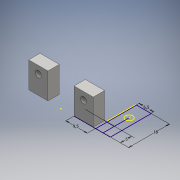
# Autodesk Inventor part: Part1
Saved by Autodesk Inventor 2016 (Build 200138000, 138)
## iProperties
Created: 2016-10-10
Part Number: Part1
Material: Generic
Document SubType Name: Modeling
Designer: yurra
Density: 1 g/cm^3
Appearance: Default
Author: yurra
Autodesk Inventor part; units mm, degrees
ref_plane "YZ Plane" through (0, 0, 0) normal (1, 0, 0) x (0, 1, 0)
ref_plane "XZ Plane" through (0, 0, 0) normal (0, 1, 0) x (-1, 0, 0)
sketch "Sketch1" plane through (0, 0, 0) normal (0, 1, 0) x (-1, 0, 0)
  line L0 (5.75, 3.75) -> (-5.75, 3.75)
  line L1 (-5.75, 3.75) -> (-5.75, -3.75)
  line L2 (-5.75, -3.75) -> (5.75, -3.75)
  line L3 (5.75, -3.75) -> (5.75, 3.75)
  line L4 (5.75, 3.75) -> (-5.75, -3.75) construction
  line L5 (-5.75, 3.75) -> (5.75, -3.75) construction
  line L6 (0, 0) -> (0, 3.75)
  circle A0 centre (10, 0.5) radius 1.25
  circle A1 centre (-10, 0.5) radius 1.25
  line L7 (8.328, 1.75) -> (12.3503, 1.75)
  line L8 (8.75, 3.0207) -> (8.75, -2.5964)
  line L9 (5.05, 3.25) -> (-5.05, 3.25)
  line L10 (-5.05, 3.25) -> (-5.05, -3.25)
  line L11 (-5.05, -3.25) -> (5.05, -3.25)
  line L12 (5.05, -3.25) -> (5.05, 3.25)
  line L13 (5.05, 3.25) -> (-5.05, -3.25) construction
  line L14 (-5.05, 3.25) -> (5.05, -3.25) construction
  dimension "d7" = 2.5
  dimension "d13" = 7.5
  dimension "d14" = 11.5
  dimension "d16" = 2
  dimension "d17" = 3
  dimension "d31" = 10.1
  dimension "d32" = 6.5
  constraints: 30 end point, 5 midpoint, 4 parallel, 3 horizontal, 2 centre point, 2 perpendicular, 2 tangent, 1 vertical, 1 other
  measures "d7" diameter of A0
  measures "d13" distance between parallel lines of L2 L0
  measures "d14" distance between parallel lines of L1 L3
  measures "d16" distance between parallel lines of L0 L7
  measures "d17" distance between parallel lines of L3 L8
  measures "d31" distance of L11.end L10.end
  measures "d32" distance of L10.end L9.end
sketch "Sketch2" plane through (0, 0, 0) normal (0, 0, 1) x (1, 0, 0)
  line L0 (0, 0) -> (0, 5)
  line L1 (0, 5) -> (0, 11.5)
  line L2 (-14.9, 5) -> (14.9, 5)
  line L3 (14.9, 5) -> (14.9, 18)
  line L4 (14.9, 18) -> (-14.9, 18)
  line L5 (-14.9, 18) -> (-14.9, 5)
  line L6 (-14.9, 5) -> (14.9, 18) construction
  line L7 (14.9, 5) -> (-14.9, 18) construction
  line L8 (0, 11.5) -> (-18.5, 11.5)
  circle A0 centre (-18.5, 11.5) radius 1.6
  circle A1 centre (18.5, 11.5) radius 1.6
  dimension "d23" = 5
  dimension "d24" = 6.5
  dimension "d25" = 29.8
  dimension "d26" = 13
  dimension "d27" = 18.5
  dimension "d28" = 3.2
  constraints: 18 end point, 2 centre point, 2 midpoint, 2 parallel, 2 perpendicular, 2 vertical, 1 coincident, 1 horizontal, 1 symmetric about line, 1 other
  measures "d23" distance of L0.start L0.end
  measures "d24" distance of L0.end L1.end
  measures "d25" distance of L4.end L3.end
  measures "d26" distance of L3.end L2.end
  measures "d27" distance of L1.end L8.end
  measures "d28" diameter of A0
ref_plane "Work Plane2" through (0, 0, -6.75) normal (0, 0, 1) x (1, 0, 0)
sketch "Sketch3" plane through (0, 0, -6.75) normal (0, 0, 1) x (1, 0, 0)
  line L0 (0, 0) -> (0, 5) projected
  line L1 (-14.9, 5) -> (14.9, 5) projected
  line L2 (-14.9, 18) -> (-14.9, 5) projected
  line L3 (0, 5) -> (0, 11.5) projected
  line L4 (0, 11.5) -> (-18.5, 11.5) projected
  circle A0 centre (-18.5, 11.5) radius 1.6 projected
  line L5 (14.9, 18) -> (-14.9, 18) projected
  line L6 (14.9, 5) -> (14.9, 18) projected
  circle A1 centre (18.5, 11.5) radius 1.6 projected
sketch "Sketch4" plane through (0, 0, 0) normal (0, 1, 0) x (-1, 0, 0)
  line L0 (-14.25, -2.75) -> (-5.75, -2.75)
  line L1 (-5.75, -2.75) -> (-5.75, 3.75)
  line L2 (-5.75, 3.75) -> (-14.25, 3.75)
  line L3 (-14.25, 3.75) -> (-14.25, -2.75)
  line L4 (-14.25, -2.75) -> (-5.75, 3.75) construction
  line L5 (-5.75, -2.75) -> (-14.25, 3.75) construction
  line L6 (0, 0) -> (0, 3.75) projected
  line L7 (14.25, -2.75) -> (5.75, -2.75)
  line L8 (5.75, -2.75) -> (5.75, 3.75)
  line L9 (5.75, 3.75) -> (14.25, 3.75)
  line L10 (14.25, 3.75) -> (14.25, -2.75)
  point P0 (-10, 0.5)
  point P1 (-10, 0.5)
  point P2 (-10, 0.5)
  point P3 (10, 0.5)
  point P4 (10, 0.5)
  constraints: 20 end point, 4 symmetric about line, 2 coincident, 2 midpoint, 2 parallel, 1 horizontal, 1 perpendicular
extrude "Extrusion1" add sketch "Sketch4" along normal blind 2.5 contours L3 L2 L1 L0
extrude "Extrusion2" add sketch "Sketch4" along normal blind 2.5 contours L7 L8 L9 L10
hole "Hole1" at (10, 0, 0.5) at (-10, 0, 0.5) direction (0, 1, 0) diameter 2.7 end through all
sketch "Sketch5" plane through (0, 2.5, 0) normal (0, 1, 0) x (1, 0, 0)
  line L0 (5.75, -3.75) -> (5.75, 2.75) projected
  line L1 (5.75, 2.75) -> (14.25, 2.75) projected
  line L2 (14.25, 2.75) -> (14.25, -3.75) projected
  line L3 (14.25, -3.75) -> (5.75, -3.75) projected
  line L4 (7.5, 1.85) -> (12.5, 1.85)
  line L5 (12.5, 1.85) -> (12.5, -2.85)
  line L6 (12.5, -2.85) -> (7.5, -2.85)
  line L7 (7.5, -2.85) -> (7.5, 1.85)
  line L8 (0, 0) -> (0, -3.75) projected
  line L9 (-5.75, -3.75) -> (-5.75, 2.75)
  line L10 (-5.75, 2.75) -> (-14.25, 2.75)
  line L11 (-14.25, 2.75) -> (-14.25, -3.75)
  line L12 (-14.25, -3.75) -> (-5.75, -3.75)
  line L13 (-7.5, 1.85) -> (-12.5, 1.85)
  line L14 (-12.5, 1.85) -> (-12.5, -2.85)
  line L15 (-12.5, -2.85) -> (-7.5, -2.85)
  line L16 (-7.5, -2.85) -> (-7.5, 1.85)
  dimension "d69" = 1.75
  dimension "d70" = 0.9
  dimension "d71" = 1.75
  dimension "d72" = 0.9
  constraints: 24 end point, 8 symmetric about line, 2 parallel, 1 horizontal, 1 perpendicular
  measures "d69" distance between parallel lines of L7 L0
  measures "d70" distance between parallel lines of L1 L4
  measures "d71" distance between parallel lines of L2 L5
  measures "d72" distance between parallel lines of L3 L6
extrude "Extrusion8" add sketch "Sketch5" along normal blind 2.5
sketch "Sketch8" plane through (14.25, 0, -2.75) normal (0, 0, -1) x (-1, 0, 0)
  line L0 (14.25, 0) -> (14.25, 5) projected
  line L1 (8.5, 0) -> (8.5, 5) projected
  line L2 (0, 5) -> (8.5, 5)
  line L3 (8.5, 5) -> (8.5, 0)
  line L4 (8.5, 0) -> (0, 0)
  line L5 (0, 0) -> (0, 5)
  line L6 (20, 0) -> (20, 5)
  line L7 (28.5, 5) -> (20, 5)
  line L8 (20, 5) -> (20, 0)
  line L9 (20, 0) -> (28.5, 0)
  line L10 (28.5, 0) -> (28.5, 5)
  constraints: 18 end point, 5 symmetric about line, 2 parallel, 1 horizontal, 1 perpendicular
extrude "Extrusion9" add sketch "Sketch8" along normal blind 5
sketch "Sketch10" plane through (14.25, 0, -7.75) normal (0, 0, -1) x (-1, 0, 0)
  circle A0 centre (-4.25, 11.5) radius 1.6 projected
  circle A1 centre (32.75, 11.5) radius 1.6 projected
  line L0 (-4.25, 11.5) -> (-4.25, 0)
  line L1 (8.5, 5) -> (0, 5) projected
  line L2 (8.5, 5) -> (-4.25, 5)
  line L3 (-4.25, 5) -> (-4.25, 0)
  line L4 (-4.25, 0) -> (8.5, 0)
  line L5 (8.5, 0) -> (8.5, 5)
  line L6 (-0.65, 5) -> (-0.65, 18) projected
  line L7 (-1, 0) -> (-1, 5)
  line L8 (-1, 0) -> (-7.5, 0)
  line L9 (-7.5, 0) -> (-7.5, 18)
  line L10 (-7.5, 18) -> (-1, 18)
  line L11 (-1, 18) -> (-1, 0)
  point P0 (14.25, 0)
  dimension "d78" = 9.5
  dimension "d79" = 5
  dimension "d80" = 6.5
  dimension "d81" = 18
  constraints: 20 end point, 4 parallel, 3 perpendicular, 2 horizontal, 2 point on line, 1 vertical
  measures "d78" distance between parallel lines of L5 L7
  measures "d79" distance between parallel lines of L4 L1
  measures "d80" distance of L9.end L10.end
  measures "d81" distance of L8.end L9.end
body "Solid1"
